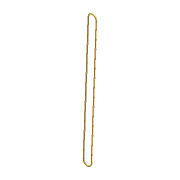
# Autodesk Inventor part: Belt_Vertical_Long2
Saved by Autodesk Inventor 2012 (Build 160160000, 160)
## iProperties
Created: 2012-01-13
Part Number: Belt_Vertical_Long2
Material: Default
Document SubType Name: Modeling
Designer: JesseK
Density: 1 g/cm^3
Mass: 37.4427 g
Surface Area: 314.36 cm^2
Volume: 37.4427 cm^3
Author: JesseK
Autodesk Inventor part; units mm, degrees
ref_plane "YZ Plane" through (0, 0, 0) normal (1, 0, 0) x (0, 1, 0)
ref_plane "XZ Plane" through (0, 0, 0) normal (0, 1, 0) x (-1, 0, 0)
ref_plane "XY Plane" through (0, 0, 0) normal (0, 0, 1) x (1, 0, 0)
sketch "Sketch1" plane through (0, 0, 0) normal (0, 0, 1) x (1, 0, 0)
  arc A0 (25.4346, -0.9988) -> (-25.4346, 0.9988) centre (0, 0) ccw
  arc A1 (-58.3107, -836.2235) -> (-7.4415, -838.2211) centre (-32.8761, -837.2223) ccw
  arc A2 (-63.0695, -836.0367) -> (-2.6827, -838.4079) centre (-32.8761, -837.2223) ccw
  arc A3 (30.1934, -1.1856) -> (-30.1934, 1.1856) centre (0, 0) ccw
  line L0 (-30.1934, 1.1856) -> (-63.0695, -836.0367)
  line L1 (-58.3107, -836.2235) -> (-25.4346, 0.9988)
  line L2 (25.4346, -0.9988) -> (-7.4415, -838.2211)
  line L3 (-2.6827, -838.4079) -> (30.1934, -1.1856)
  dimension "d0" = 4.7625
  constraints: 8 end point, 8 point on circle, 8 tangent, 4 centre point, 3 coincident, 2 parallel
  measures "d0" radial gap between concentric circles of A2 A1
extrude "Extrusion1" add sketch "Sketch1" along normal blind 4.7625
fillet "Fillet1" radius 2.3813 8 edges at (-34.0618, -867.4157, 4.7625) (-46.6315, -417.4255, 4.7625) (1.1856, 30.1934, 4.7625) (13.7554, -419.7968, 4.7625) (1.1856, 30.1934, 0) (-46.6315, -417.4255, 0) (-34.0618, -867.4157, 0) (13.7554, -419.7968, 0)
body "Solid1"
